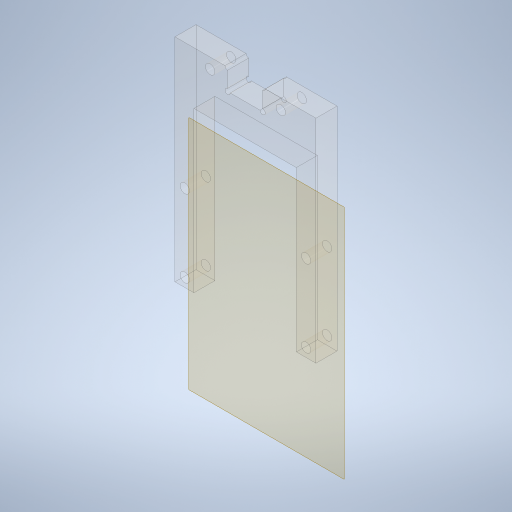
# Autodesk Inventor part: feet_holder2
Saved by Autodesk Inventor 2024 (Build 280153000, 153)
## iProperties
Created: 2024-09-03
Part Number: feet_holder2
Material: PMMA 플라스틱
Document SubType Name: Modeling
Designer: jmha0
Density: 1.188 g/cm^3
Appearance: 폴리카보네이트 - 선명
Mass: 7.49643 g
Surface Area: 42.8866 cm^2
Volume: 6.31012 cm^3
Author: jmha0
Autodesk Inventor part; units mm, degrees
ref_plane "YZ Plane" through (0, 0, 0) normal (1, 0, 0) x (0, 1, 0)
ref_plane "XZ Plane" through (0, 0, 0) normal (0, 1, 0) x (-1, 0, 0)
ref_plane "XY Plane" through (0, 0, 0) normal (0, 0, 1) x (1, 0, 0)
ref_plane "작업 평면1" through (0, 0, 0) normal (0, 0, 1) x (1, 0, 0)
sketch "스케치1" plane through (0, 0, 0) normal (0, 0, 1) x (1, 0, 0)
  line L0 (14.5, -41) -> (14.5, 11) projected
  line L1 (20.1, -39.6766) -> (20.1, 4.5766) projected
  line L2 (-20.1, 4.5766) -> (-20.1, -39.6766) projected
  line L3 (-14.5, 11) -> (-14.5, -41) projected
  circle A0 centre (-17.3, -18) radius 1.35 projected
  circle A1 centre (17.3, -18) radius 1.35 projected
  circle A2 centre (17.3, 4) radius 1.35 projected
  circle A3 centre (-17.3, 4) radius 1.35 projected
  circle A4 centre (17.3, -18) radius 1.45
  circle A5 centre (-17.3, -18) radius 1.45
  circle A6 centre (-17.3, 4) radius 1.45
  circle A7 centre (17.3, 4) radius 1.45
  line L4 (14.7, -41) -> (14.7, 11)
  line L5 (-14.7, 11) -> (-14.7, -41)
  line L6 (20.1, -20.5011) -> (-20.1, -20.5011)
  line L7 (-20.1, 0) -> (-20.1, 40)
  line L8 (20.1, -20.5011) -> (20.1, 40)
  line L9 (20.1, 40) -> (-20.1, 40)
  line L10 (14.5, 0) -> (14.5, 25)
  line L11 (14.5, 25) -> (-14.7, 25)
  line L12 (-14.7, 25) -> (-14.7, 0)
  line L13 (20.1, 40) -> (15.1, 40)
  line L14 (20.1, 40) -> (10.05, 40)
  line L15 (10.05, 40) -> (0, 40)
  line L16 (0, 40) -> (-10.05, 40)
  line L17 (-10.05, 40) -> (-20.1, 40)
  line L18 (20.1, 25) -> (20.1, 32.5)
  circle A8 centre (10.05, 32.5) radius 1.4
  circle A9 centre (-10.05, 32.5) radius 1.4
  point P0 (0, 0)
  point P1 (0, -20.5011)
  point P2 (-14.7, -20.5011)
  point P3 (14.5, -20.5011)
  dimension "d0" = 0.1
  dimension "d1" = 0.1
  dimension "d2" = -0.1
  dimension "d3" = 0.1
  dimension "d4" = 0.2
  dimension "d5" = 0.2
  dimension "d6" = 20.5011
  dimension "d7" = 40
  dimension "d9" = 15
  dimension "d12" = 5
  dimension "d13" = 40.2
  dimension "d14" = 10.05
  dimension "d15" = 10.05
  dimension "d16" = 10.05
  dimension "d17" = 10.05
  dimension "d18" = 7.5
  dimension "d19" = 2.8
  dimension "d20" = 2.8
  dimension "d21" = 20.1
  constraints: 30 end point, 10 point on line, 6 centre point, 3 perpendicular, 3 vertical, 2 midpoint, 2 parallel, 1 collinear
  measures "d0" radial gap between concentric circles of A1 A4
  measures "d1" radial gap between concentric circles of A0 A5
  measures "d2" radial gap between concentric circles of A3 A6
  measures "d3" radial gap between concentric circles of A2 A7
  measures "d4" distance between parallel lines of L0 L4
  measures "d5" distance between parallel lines of L3 L5
  measures "d6" distance of point (0, -20.501) point (0, 0)
  measures "d7" distance of L7.start L7.end
  measures "d9" distance between parallel lines of L9 L11
  measures "d12" distance of L8.end L13.end
  measures "d13" distance between parallel lines of L7 L8
  measures "d14" distance of L8.end L14.end
  measures "d15" distance of L14.end L15.end
  measures "d16" distance of L15.end L16.end
  measures "d17" distance of L16.end L7.end
  measures "d18" distance of L18.start L18.end
  measures "d19" diameter of A8
  measures "d20" diameter of A9
  measures "d21" distance of A9.centre A8.centre
extrude "돌출1" add sketch "스케치1" along normal blind 6 contours L0 L10 L11 L12 L5 L6 L2 L7 L9 L8 L1 | A4 | A5 | A6 | A7 | A8 | A9
sketch "스케치3" plane through (-20.1, 40, 0) normal (0, 1, 0) x (1, 0, 0)
  line L0 (40.2, 0) -> (0, 0) projected
  line L1 (0, 0) -> (0, -6) projected
  line L2 (40.2, -6) -> (0, -6) projected
  line L3 (40.2, 0) -> (40.2, -6) projected
  point P0 (20.1, 0)
  dimension "d29" = 40.2
  measures "d29" distance of L0.start L0.end
sketch "스케치4" plane through (0, 0, 6) normal (0, 0, 1) x (1, 0, 0)
  line L0 (20.1, 40) -> (-20.1, 40) projected
  line L1 (-20.1, 40) -> (20.1, 40)
  line L2 (20.1, 40) -> (20.1, 34)
  line L3 (20.1, 34) -> (-20.1, 34)
  line L4 (-20.1, 34) -> (-20.1, 40)
  line L5 (-20.1, 40) -> (-10.05, 40)
  line L6 (-10.05, 40) -> (10.05, 40)
  circle A0 centre (-10.05, 37) radius 1.35
  circle A1 centre (10.05, 37) radius 1.35
  point P0 (0, 0)
  dimension "d30" = 6
  dimension "d31" = 10.05
  dimension "d32" = 20.1
  dimension "d33" = 2.7
  dimension "d34" = 2.7
  constraints: 12 end point, 3 equal length, 2 centre point, 2 point on line, 1 perpendicular
  measures "d30" distance of L0.start L2.end
  measures "d31" distance of L0.end L5.end
  measures "d32" distance of L5.end L6.end
  measures "d33" diameter of A0
  measures "d34" diameter of A1
extrude "돌출3" cut sketch "스케치4" against normal blind 10 contours A0 | A1
sketch "스케치5" plane through (0, 0, 6) normal (0, 0, 1) x (1, 0, 0)
  circle A0 centre (10.05, 37) radius 1.35 projected
  circle A1 centre (-10.05, 37) radius 1.35 projected
  line L0 (14.5, 25) -> (14.5, -20.5011) projected
  line L1 (14.5, -20.5011) -> (20.1, -20.5011) projected
  line L2 (20.1, -20.5011) -> (20.1, 40) projected
  line L3 (20.1, 40) -> (-20.1, 40) projected
  line L4 (-20.1, 40) -> (-20.1, -20.5011) projected
  line L5 (-20.1, -20.5011) -> (-14.7, -20.5011) projected
  line L6 (-14.7, -20.5011) -> (-14.7, 25) projected
  line L7 (-14.7, 25) -> (14.5, 25) projected
  circle A2 centre (17.3, 4) radius 1.35 projected
  circle A3 centre (17.3, -18) radius 1.35 projected
  circle A4 centre (-17.3, -18) radius 1.35 projected
  circle A5 centre (-17.3, 4) radius 1.35 projected
  line L8 (4.9, 34) -> (-5.1, 34)
  line L9 (-5.1, 34) -> (-5.1, 40)
  line L10 (-5.1, 40) -> (4.9, 40)
  line L11 (4.9, 40) -> (4.9, 34)
  line L12 (4.9, 34) -> (-5.1, 40) construction
  line L13 (-5.1, 34) -> (4.9, 40) construction
  circle A6 centre (-5.1, 40) radius 0.75
  circle A7 centre (-5.1, 34) radius 0.75
  circle A8 centre (4.9, 34) radius 0.75
  circle A9 centre (4.9, 40) radius 0.75
  point P0 (0, 0)
  point P1 (-0.1, 37)
  point P2 (4.15, 34)
  point P3 (4.9, 34.75)
  point P4 (-5.1, 34.75)
  point P5 (-4.35, 34)
  point P6 (-5.1, 39.25)
  point P7 (-4.35, 40)
  point P8 (4.9, 39.25)
  point P9 (5.65, 40)
  dimension "d37" = 10
  dimension "d40" = 1.5
  dimension "d41" = 1.5
  dimension "d42" = 1.5
  dimension "d43" = 1.5
  constraints: 12 end point, 4 centre point, 4 coincident, 2 midpoint, 2 parallel, 1 horizontal, 1 perpendicular, 1 point on line
  measures "d37" distance of L9.end L10.end
  measures "d40" diameter of A6
  measures "d41" diameter of A7
  measures "d42" diameter of A8
  measures "d43" diameter of A9
extrude "돌출4" cut sketch "스케치5" against normal blind 6 contours A9 L11 L3 | L11 A9 L3 | A9 L11 A8 L8 A7 L9 A6 L3 | A6 L3 | L3 L9 A6 | A6 L9 L3 | A8 L8 L11 | L11 L8 A8 | A7 L8 L9 | L9 L8 A7
